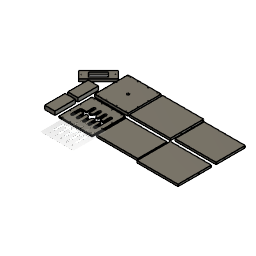
H shifeter (Autodesk Fusion 360 design; units mm, degrees)
part number: 2026-02-17-17-36-58-814
Autodesk Fusion 360 part; units mm, degrees
sketch "Sketch2" plane through (0, 0, 0) normal (0, 1, 0) x (1, 0, 0)
  line L0 (0, 65) -> (-65, 65)
  line L1 (-65, 65) -> (65, 65)
  line L2 (65, 65) -> (65, -65)
  line L3 (65, -65) -> (-65, -65)
  line L4 (-65, -65) -> (-65, 65)
  circle A0 centre (0, 0) radius 4.5
  circle A1 centre (-61, -63) radius 1
  circle A2 centre (-61, 61) radius 1
  circle A3 centre (-61, 17) radius 1
  circle A4 centre (-61, -23) radius 1
  line L5 (100, -65) -> (108, -65)
  line L6 (108, -65) -> (108, 65)
  line L7 (108, 65) -> (100, 65)
  line L8 (100, 65) -> (100, -65)
  line L9 (104, -64) -> (104, -63)
  line L10 (104, -63) -> (103, -63)
  circle A5 centre (104, -63) radius 1
  circle A6 centre (104, -23) radius 1
  circle A7 centre (104, 17) radius 1
  circle A8 centre (104, 61) radius 1
  line L11 (108, -65) -> (108, 65)
  line L12 (100, 65) -> (100, -65)
  line L13 (108, -65) -> (108, 65)
  line L14 (108, -65) -> (108, 65)
  circle A9 centre (104, -63) radius 1
  line L15 (104, -64) -> (104, -63)
  line L16 (100, -65) -> (108, -65)
  circle A10 centre (104, 61) radius 1
  line L17 (100, 65) -> (100, -65)
  circle A11 centre (104, -23) radius 1
  circle A12 centre (104, 17) radius 1
  line L18 (108, 65) -> (100, 65)
  line L19 (100, 65) -> (100, -65)
  line L20 (198, -57) -> (198, 57)
  line L21 (194, 52) -> (194, 54)
  line L22 (194, 52) -> (194, 54)
  line L23 (194, 52) -> (194, 53)
  line L24 (190, 57) -> (190, -57)
  line L25 (198, -57) -> (198, 57)
  line L26 (190, 57) -> (190, -57)
  line L27 (190, 57) -> (190, -57)
  circle A13 centre (61, -63) radius 1
  line L28 (65, -65) -> (65, 65)
  line L29 (65, -65) -> (65, 65)
  circle A14 centre (61, -63) radius 1
  line L30 (65, -65) -> (65, 65)
  line L31 (61, -65) -> (61, -63)
  circle A15 centre (61, -23) radius 1
  circle A16 centre (61, -23) radius 1
  line L32 (61, -63) -> (60, -63)
  line L33 (65, -65) -> (65, 65)
  line L34 (57, -65) -> (65, -65)
  circle A17 centre (61, 17) radius 1
  line L35 (61, -65) -> (61, -63)
  line L36 (61, -63) -> (60, -63)
  line L37 (57, -65) -> (65, -65)
  line L38 (65, 65) -> (57, 65)
  line L39 (65, 65) -> (57, 65)
  circle A18 centre (61, 61) radius 1
  circle A19 centre (61, 17) radius 1
  circle A20 centre (61, 61) radius 1
  line L40 (65, 57) -> (65, 65)
  circle A21 centre (17, 61) radius 1
  line L41 (-65, 65) -> (-65, 57)
  circle A22 centre (17, 61) radius 1
  circle A23 centre (61, 61) radius 1
  line L42 (65, 57) -> (65, 65)
  line L43 (-65, 65) -> (-65, 57)
  line L44 (65, 65) -> (-65, 65)
  line L45 (65, 65) -> (-65, 65)
  line L46 (65, 65) -> (-65, 65)
  line L47 (65, 65) -> (-65, 65)
  circle A24 centre (-23, 61) radius 1
  circle A25 centre (-23, 61) radius 1
  circle A26 centre (53, 61) radius 1
  line L48 (190, 57) -> (198, 57)
  line L49 (194, 54) -> (194, 53)
  circle A27 centre (194, 53) radius 1
  line L50 (190, -57) -> (198, -57)
  line L51 (190, 57) -> (190, -57)
  line L52 (194, -54) -> (194, -52)
  line L53 (194, -54) -> (194, -53)
  circle A28 centre (194, -53) radius 1
  circle A29 centre (-53, 61) radius 1
  circle A30 centre (194, -23) radius 1
  line L54 (194, -23) -> (194, -22)
  line L55 (194, 52) -> (194, 53)
  line L56 (194, 54) -> (194, 52)
  line L57 (194, -54) -> (194, -52)
  line L58 (194, -24) -> (194, -23)
  line L59 (194, -53) -> (194, -52)
  line L60 (194, -24) -> (194, -23)
  line L61 (194, -22) -> (194, -24)
  line L62 (194, -52) -> (194, -54)
  circle A31 centre (194, 17) radius 1
  line L63 (194, -23) -> (194, -22)
  line L64 (194, 16) -> (194, 17)
  circle A32 centre (234, 53) radius 1
  line L65 (238, -57) -> (238, 57)
  circle A33 centre (234, 17) radius 1
  line L66 (234, 52) -> (234, 53)
  line L67 (234, -54) -> (234, -52)
  circle A34 centre (234, -53) radius 1
  line L68 (234, -54) -> (234, -53)
  line L69 (234, -22) -> (234, -24)
  line L70 (234, -23) -> (234, -22)
  line L71 (234, -52) -> (234, -54)
  line L72 (234, 52) -> (234, 53)
  line L73 (234, 16) -> (234, 17)
  line L74 (234, -54) -> (234, -52)
  line L75 (234, -24) -> (234, -23)
  line L76 (234, -24) -> (234, -23)
  line L77 (230, 57) -> (230, -57)
  line L78 (230, -57) -> (238, -57)
  circle A35 centre (234, -23) radius 1
  line L79 (234, -23) -> (234, -22)
  line L80 (234, 54) -> (234, 53)
  line L81 (234, -53) -> (234, -52)
  line L82 (238, -57) -> (238, 57)
  line L83 (234, 52) -> (234, 54)
  line L84 (234, 54) -> (234, 52)
  line L85 (230, 57) -> (238, 57)
  line L86 (234, 52) -> (234, 54)
  line L87 (230, 57) -> (230, -57)
  line L88 (230, 57) -> (230, -57)
  line L89 (230, 57) -> (230, -57)
  line L90 (-24, -61) -> (-23, -61)
  line L91 (-24, -61) -> (-23, -61)
  line L92 (-52, -61) -> (-54, -61)
  line L93 (-22, -61) -> (-24, -61)
  line L94 (-23, -61) -> (-22, -61)
  circle A36 centre (-23, -61) radius 1
  line L95 (-23, -61) -> (-22, -61)
  line L96 (-54, -61) -> (-53, -61)
  circle A37 centre (17, -61) radius 1
  line L97 (52, -61) -> (53, -61)
  line L98 (52, -61) -> (54, -61)
  line L99 (-53, -61) -> (-52, -61)
  line L100 (52, -61) -> (53, -61)
  circle A38 centre (53, -61) radius 1
  line L101 (54, -61) -> (53, -61)
  line L102 (52, -61) -> (54, -61)
  line L103 (54, -61) -> (52, -61)
  line L104 (-54, -61) -> (-52, -61)
  line L105 (-54, -61) -> (-52, -61)
  circle A39 centre (-53, -61) radius 1
  line L106 (16, -61) -> (17, -61)
  line L107 (-61, -63) -> (-61, -62)
  line L108 (-61, -24) -> (-61, -23)
  line L109 (-61, -23) -> (-61, -22)
  line L110 (-61, 16) -> (-61, 17)
  line L111 (-61, 17) -> (-61, 18)
  line L112 (-61, 60) -> (-61, 61)
  line L113 (-24, 61) -> (-23, 61)
  line L114 (-24, 61) -> (-23, 61)
  line L115 (-62, 61) -> (-60, 61)
  line L116 (-57, 61) -> (-52, 61)
  line L117 (-62, 61) -> (-60, 61)
  line L118 (-54, 61) -> (-52, 61)
  line L119 (-23, 61) -> (-22, 61)
  line L120 (16, 61) -> (17, 61)
  line L121 (-23, 61) -> (-22, 61)
  line L122 (16, 61) -> (17, 61)
  line L123 (17, 61) -> (18, 61)
  line L124 (17, 61) -> (18, 61)
  line L125 (17, 61) -> (18, 61)
  line L126 (17, 61) -> (18, 61)
  line L127 (60, 61) -> (61, 61)
  line L128 (52, 61) -> (54, 61)
  line L129 (60, 61) -> (61, 61)
  line L130 (52, 61) -> (54, 61)
  line L131 (60, 61) -> (61, 61)
  line L132 (52, 61) -> (54, 61)
  line L133 (60, 61) -> (61, 61)
  line L134 (61, 17) -> (61, 18)
  line L135 (61, 60) -> (61, 61)
  line L136 (61, 17) -> (61, 18)
  line L137 (61, 60) -> (61, 61)
  line L138 (61, 17) -> (61, 18)
  line L139 (61, 60) -> (61, 61)
  line L140 (61, 17) -> (61, 18)
  line L141 (61, 60) -> (61, 61)
  line L142 (61, -23) -> (61, -22)
  line L143 (61, 16) -> (61, 17)
  line L144 (61, -23) -> (61, -22)
  line L145 (61, 16) -> (61, 17)
  line L146 (61, -63) -> (61, -62)
  line L147 (61, -24) -> (61, -23)
  line L148 (61, -63) -> (61, -62)
  line L149 (61, -24) -> (61, -23)
  line L150 (104, -23) -> (104, -22)
  line L151 (104, 16) -> (104, 17)
  line L152 (104, -63) -> (104, -62)
  line L153 (104, -24) -> (104, -23)
  line L154 (104, -23) -> (104, -22)
  line L155 (104, 16) -> (104, 17)
  line L156 (104, -63) -> (104, -62)
  line L157 (104, -24) -> (104, -23)
  line L158 (104, 17) -> (104, 18)
  line L159 (104, 60) -> (104, 61)
  line L160 (104, 17) -> (104, 18)
  line L161 (104, 60) -> (104, 61)
  line L162 (104, 17) -> (104, 18)
  line L163 (104, 60) -> (104, 61)
  line L164 (104, 17) -> (104, 18)
  line L165 (104, 60) -> (104, 61)
  circle A40 centre (134, -23) radius 1
  line L166 (138, -65) -> (138, 65)
  line L167 (138, -65) -> (138, 65)
  line L168 (138, -65) -> (138, 65)
  line L169 (134, -24) -> (134, -23)
  line L170 (134, -23) -> (134, -22)
  line L171 (130, 65) -> (130, -65)
  line L172 (138, -65) -> (138, 65)
  line L173 (130, 65) -> (130, -65)
  circle A41 centre (134, 61) radius 1
  line L174 (134, 17) -> (134, 18)
  line L175 (138, 65) -> (130, 65)
  line L176 (134, 60) -> (134, 61)
  line L177 (134, 17) -> (134, 18)
  circle A42 centre (134, 17) radius 1
  line L178 (134, 17) -> (134, 18)
  circle A43 centre (134, 61) radius 1
  line L179 (134, 60) -> (134, 61)
  circle A44 centre (134, 17) radius 1
  line L180 (134, 60) -> (134, 61)
  line L181 (134, 60) -> (134, 61)
  line L182 (134, 16) -> (134, 17)
  line L183 (138, 65) -> (130, 65)
  circle A45 centre (134, -63) radius 1
  line L184 (130, 65) -> (130, -65)
  line L185 (130, 65) -> (130, -65)
  line L186 (134, -63) -> (133, -63)
  line L187 (134, 17) -> (134, 18)
  line L188 (134, -64) -> (134, -63)
  line L189 (134, -63) -> (134, -62)
  circle A46 centre (134, -63) radius 1
  line L190 (130, -65) -> (138, -65)
  line L191 (134, -64) -> (134, -63)
  line L192 (134, -63) -> (134, -62)
  line L193 (134, -63) -> (133, -63)
  line L194 (134, 16) -> (134, 17)
  line L195 (130, -65) -> (138, -65)
  circle A47 centre (134, -23) radius 1
  line L196 (134, -24) -> (134, -23)
  line L197 (134, -23) -> (134, -22)
  line L198 (-57, -189) -> (-52, -189)
  line L199 (16, -189) -> (17, -189)
  line L200 (-61, -234) -> (-61, -233)
  line L201 (-24, -189) -> (-23, -189)
  line L202 (-61, -233) -> (-61, -232)
  line L203 (-65, -185) -> (-65, -193)
  line L204 (-65, -185) -> (-65, -193)
  line L205 (-62, -189) -> (-60, -189)
  line L206 (-61, -190) -> (-61, -189)
  line L207 (-23, -189) -> (-22, -189)
  circle A48 centre (17, -189) radius 1
  line L208 (-62, -189) -> (-60, -189)
  circle A49 centre (-23, -189) radius 1
  line L209 (17, -189) -> (18, -189)
  line L210 (17, -189) -> (18, -189)
  line L211 (0, -185) -> (-65, -185)
  line L212 (-23, -189) -> (-22, -189)
  line L213 (17, -189) -> (18, -189)
  circle A50 centre (17, -189) radius 1
  line L214 (-54, -189) -> (-52, -189)
  line L215 (-24, -189) -> (-23, -189)
  line L216 (17, -189) -> (18, -189)
  line L217 (65, -185) -> (-65, -185)
  line L218 (-65, -185) -> (65, -185)
  line L219 (65, -185) -> (-65, -185)
  line L220 (65, -315) -> (-65, -315)
  line L221 (65, -185) -> (-65, -185)
  line L222 (65, -185) -> (-65, -185)
  line L223 (-65, -315) -> (-65, -185)
  circle A51 centre (-23, -311) radius 1
  line L224 (65, -315) -> (65, -185)
  line L225 (16, -311) -> (17, -311)
  line L226 (-53, -311) -> (-52, -311)
  line L227 (-52, -311) -> (-54, -311)
  line L228 (-23, -311) -> (-22, -311)
  line L229 (-24, -311) -> (-23, -311)
  line L230 (65, -185) -> (65, -315)
  line L231 (-22, -311) -> (-24, -311)
  circle A52 centre (-53, -311) radius 1
  line L232 (-61, -274) -> (-61, -273)
  circle A53 centre (-61, -233) radius 1
  line L233 (-54, -311) -> (-53, -311)
  circle A54 centre (-53, -189) radius 1
  circle A55 centre (-61, -273) radius 1
  line L234 (16, -189) -> (17, -189)
  circle A56 centre (-61, -313) radius 1
  line L235 (-23, -311) -> (-22, -311)
  line L236 (-61, -273) -> (-61, -272)
  line L237 (-61, -313) -> (-61, -312)
  line L238 (-54, -311) -> (-52, -311)
  circle A57 centre (17, -311) radius 1
  line L239 (-54, -311) -> (-52, -311)
  line L240 (-24, -311) -> (-23, -311)
  circle A58 centre (-23, -189) radius 1
  circle A59 centre (-61, -189) radius 1
  line L241 (65, -315) -> (65, -185)
  circle A60 centre (61, -313) radius 1
  line L242 (57, -315) -> (65, -315)
  line L243 (52, -311) -> (54, -311)
  line L244 (61, -313) -> (60, -313)
  line L245 (52, -311) -> (54, -311)
  line L246 (61, -313) -> (60, -313)
  line L247 (54, -311) -> (52, -311)
  line L248 (65, -315) -> (65, -185)
  circle A61 centre (53, -311) radius 1
  line L249 (65, -315) -> (65, -185)
  line L250 (65, -193) -> (65, -185)
  line L251 (61, -274) -> (61, -273)
  line L252 (61, -233) -> (61, -232)
  circle A62 centre (61, -273) radius 1
  circle A63 centre (61, -313) radius 1
  circle A64 centre (61, -273) radius 1
  circle A65 centre (61, -189) radius 1
  circle A66 centre (61, -233) radius 1
  line L253 (52, -189) -> (54, -189)
  line L254 (61, -234) -> (61, -233)
  line L255 (61, -190) -> (61, -189)
  line L256 (52, -189) -> (54, -189)
  line L257 (65, -193) -> (65, -185)
  line L258 (61, -274) -> (61, -273)
  line L259 (61, -313) -> (61, -312)
  line L260 (57, -315) -> (65, -315)
  line L261 (61, -233) -> (61, -232)
  line L262 (54, -311) -> (53, -311)
  line L263 (61, -233) -> (61, -232)
  line L264 (61, -273) -> (61, -272)
  line L265 (52, -189) -> (54, -189)
  circle A67 centre (61, -233) radius 1
  line L266 (65, -185) -> (57, -185)
  line L267 (52, -311) -> (53, -311)
  line L268 (61, -315) -> (61, -313)
  line L269 (61, -315) -> (61, -313)
  line L270 (65, -185) -> (57, -185)
  line L271 (52, -311) -> (53, -311)
  line L272 (61, -313) -> (61, -312)
  line L273 (60, -189) -> (61, -189)
  line L274 (60, -189) -> (61, -189)
  circle A68 centre (53, -189) radius 1
  circle A69 centre (61, -189) radius 1
  line L275 (61, -273) -> (61, -272)
  line L276 (60, -189) -> (61, -189)
  circle A70 centre (61, -189) radius 1
  line L277 (61, -233) -> (61, -232)
  line L278 (61, -190) -> (61, -189)
  line L279 (61, -190) -> (61, -189)
  line L280 (60, -189) -> (61, -189)
  line L281 (61, -190) -> (61, -189)
  line L282 (61, -234) -> (61, -233)
  arc A71 (17.3155, -282.4056) -> (26.3155, -282.4056) centre (21.8155, -282.4056) ccw
  line L283 (39, -245.5) -> (26.3155, -245.5)
  line L284 (26.3155, -254.5058) -> (39, -254.5058)
  arc A72 (48, -220) -> (39, -220) centre (43.5, -220) ccw
  arc A73 (26.3155, -220) -> (17.3155, -220) centre (21.8155, -220) ccw
  arc A74 (39, -282.4056) -> (48, -282.4056) centre (43.5, -282.4056) ccw
  line L285 (5.3081, -282.4056) -> (5.3081, -259.4163)
  arc A75 (-16.9818, -220) -> (-25.9818, -220) centre (-21.4818, -220) ccw
  line L286 (-4.241, -240.0573) -> (-4.241, -220)
  line L287 (39, -254.5058) -> (39, -282.4056)
  arc A76 (4.759, -220) -> (-4.241, -220) centre (0.259, -220) ccw
  line L288 (-18, -282.6168) -> (-18, -254.8691)
  line L289 (17.3155, -254.5058) -> (17.3155, -282.4056)
  line L290 (-27, -255) -> (-27, -282.6168)
  arc A77 (-41.9906, -245.6112) -> (-49, -251.5257) centre (-43, -251.5257) ccw
  line L291 (48, -254.5058) -> (48, -220)
  line L292 (39, -220) -> (39, -245.5)
  arc A78 (-49, -282.6168) -> (-40, -282.6168) centre (-44.5, -282.6168) ccw
  line L293 (-16.9818, -220) -> (-16.9818, -245.8691)
  arc A79 (5.3081, -259.4163) -> (9.8255, -254.5058) centre (0, -250) ccw
  line L294 (26.3155, -282.4056) -> (26.3155, -254.5058)
  line L295 (9.8255, -254.5058) -> (17.3155, -254.5058)
  arc A80 (-4.241, -240.0573) -> (-9.9889, -245.8691) centre (0, -250) ccw
  line L296 (-3.6919, -260.1594) -> (-3.6919, -282.4056)
  line L297 (-49, -282.6168) -> (-49, -251.5257)
  line L298 (17.3155, -220) -> (17.3155, -245.4147)
  line L299 (-16.9818, -245.8691) -> (-9.9889, -245.8691)
  line L300 (-8.9707, -254.8691) -> (-18, -254.8691)
  arc A81 (-27, -282.6168) -> (-18, -282.6168) centre (-22.5, -282.6168) ccw
  line L301 (-40, -255) -> (-40, -282.6168)
  line L302 (17.3155, -245.4147) -> (9.7887, -245.4147)
  line L303 (48, -282.4056) -> (48, -254.5058)
  line L304 (26.3155, -245.5) -> (26.3155, -220)
  line L305 (-27, -255) -> (-40, -255)
  arc A82 (-9.6507, -254.8691) -> (-3.6919, -260.1594) centre (0, -250) ccw
  line L306 (-25.9818, -245.6112) -> (-25.9818, -220)
  arc A83 (-3.6919, -282.4056) -> (5.3081, -282.4056) centre (0.8081, -282.4056) ccw
  arc A84 (9.7887, -245.4147) -> (4.759, -240.2946) centre (0, -250) ccw
  line L307 (4.759, -220) -> (4.759, -241)
  line L308 (-41.9906, -245.6112) -> (-25.9818, -245.6112)
  dimension "d5" = 130
  dimension "d6" = 130
  dimension "d11" = 9
  dimension "d17" = 40
  dimension "d18" = 40
  dimension "d19" = 44
  dimension "d20" = 2
  dimension "d21" = 2
  dimension "d22" = 2
  dimension "d23" = 8
  dimension "d24" = 130
  dimension "d25" = 40
  dimension "d26" = 40
  dimension "d27" = 44
  dimension "d28" = 2
  dimension "d29" = 2
  dimension "d30" = 2
  dimension "d31" = 2
  dimension "d32" = 8
  dimension "d33" = 130
  dimension "d34" = 44
  dimension "d45" = 8
  dimension "d46" = 130
  dimension "d47" = 40
  dimension "d48" = 40
  dimension "d49" = 44
  dimension "d50" = 2
  dimension "d51" = 2
  dimension "d52" = 2
  dimension "d53" = 2
  dimension "d54" = 8
  dimension "d55" = 130
  dimension "d56" = 44
  dimension "d111" = 8
  dimension "d112" = 130
  dimension "d113" = 40
  dimension "d114" = 40
  dimension "d115" = 44
  dimension "d116" = 2
  dimension "d117" = 2
  dimension "d118" = 2
  dimension "d119" = 2
  dimension "d122" = 44
  dimension "d123" = 8
  dimension "d124" = 130
  dimension "d125" = 40
  dimension "d126" = 40
  dimension "d127" = 44
  dimension "d128" = 2
  dimension "d129" = 2
  dimension "d130" = 2
  dimension "d131" = 2
  dimension "d134" = 44
  dimension "d135" = 8
  dimension "d136" = 130
  dimension "d138" = 40
  dimension "d139" = 44
  dimension "d141" = 2
  dimension "d142" = 2
  dimension "d143" = 2
  dimension "d145" = 130
  dimension "d146" = 44
  dimension "d147" = 8
  dimension "d148" = 130
  dimension "d150" = 40
  dimension "d151" = 44
  dimension "d153" = 2
  dimension "d154" = 2
  dimension "d157" = 130
  dimension "d158" = 44
  dimension "d159" = 2
  dimension "d162" = 2
  dimension "d164" = 2
  dimension "d166" = 2
  dimension "d167" = 30
  dimension "d168" = 2
  dimension "d171" = 40
  dimension "d172" = 2
  dimension "d173" = 2
  dimension "d174" = 2
  dimension "d175" = 30
  dimension "d176" = 2
  dimension "d177" = 40
  dimension "d178" = 2
  dimension "d179" = 2
  dimension "d180" = 2
  dimension "d181" = 30
  dimension "d182" = 2
  dimension "d183" = 40
  dimension "d184" = 2
  dimension "d185" = 8
  dimension "d186" = 130
  dimension "d187" = 40
  dimension "d188" = 40
  dimension "d189" = 44
  dimension "d190" = 2
  dimension "d191" = 2
  dimension "d192" = 2
  dimension "d193" = 2
  dimension "d194" = 8
  dimension "d195" = 130
  dimension "d196" = 44
  dimension "d197" = 8
  dimension "d198" = 130
  dimension "d199" = 40
  dimension "d200" = 40
  dimension "d201" = 44
  dimension "d202" = 2
  dimension "d203" = 2
  dimension "d204" = 2
  dimension "d205" = 2
  dimension "d206" = 8
  dimension "d207" = 130
  dimension "d208" = 44
  dimension "d209" = 130
  dimension "d210" = 130
  dimension "d212" = 40
  dimension "d213" = 40
  dimension "d214" = 44
  dimension "d215" = 2
  dimension "d216" = 2
  dimension "d217" = 2
  dimension "d218" = 8
  dimension "d219" = 130
  dimension "d220" = 40
  dimension "d221" = 40
  dimension "d222" = 44
  dimension "d223" = 2
  dimension "d224" = 2
  dimension "d225" = 2
  dimension "d226" = 2
  dimension "d227" = 44
  dimension "d228" = 8
  dimension "d229" = 130
  dimension "d230" = 40
  dimension "d231" = 40
  dimension "d232" = 44
  dimension "d233" = 2
  dimension "d234" = 2
  dimension "d235" = 2
  dimension "d236" = 2
  dimension "d237" = 44
  dimension "d238" = 8
  dimension "d239" = 130
  dimension "d240" = 40
  dimension "d241" = 44
  dimension "d242" = 2
  dimension "d243" = 2
  dimension "d244" = 2
  dimension "d245" = 130
  dimension "d246" = 44
  dimension "d247" = 8
  dimension "d248" = 130
  dimension "d249" = 40
  dimension "d250" = 44
  dimension "d251" = 2
  dimension "d252" = 2
  dimension "d253" = 130
  dimension "d254" = 44
  dimension "d255" = 2
  dimension "d256" = 2
  dimension "d257" = 2
  dimension "d258" = 2
  dimension "d259" = 30
  dimension "d260" = 2
  dimension "d261" = 40
  dimension "d262" = 2
  dimension "d274" = 9
  dimension "d275" = 9
  dimension "d276" = 9
  dimension "d277" = 9
  dimension "d278" = 9
  dimension "d279" = 9
  dimension "d280" = 25.5
  dimension "d281" = 9
  dimension "d282" = 9
  dimension "d283" = 9
  constraint horizontal L1
  constraint vertical L2
  constraint horizontal L3
  constraint vertical L4
  constraint coincident A0.centre origin
  constraint coincident A1.centre L107.start
  constraint parallel L4 L107
  constraint parallel L108 L109
  constraint parallel L110 L111
  constraint coincident A2.centre L112.end
  constraint coincident A3.centre L110.end
  constraint coincident A4.centre L108.end
  constraint horizontal L5
  constraint vertical L6
  constraint horizontal L7
  constraint vertical L8
  constraint perpendicular L5 L9
  constraint perpendicular L8 L10
  constraint perpendicular L10 L156
  constraint perpendicular L10 L150
  constraint perpendicular L10 L162
  constraint coincident L9.end L10.start
  constraint coincident A6.centre A11.centre
  constraint coincident A7.centre A12.centre
  constraint coincident A8.centre A10.centre
  constraint vertical L11
  constraint vertical L12
  constraint horizontal L16
  constraint vertical L13
  constraint horizontal L18
  constraint vertical L19
  constraint perpendicular L15 L16
  constraint vertical L14
  constraint vertical L17
  constraint vertical L25
  constraint vertical L51
  constraint vertical L24
  constraint vertical L27
  constraint vertical L20
  constraint vertical L26
  constraint horizontal L37
  constraint vertical L33
  constraint horizontal L39
  constraint midpoint L31.start L37
  constraint perpendicular L31 L37
  constraint perpendicular L36 L148
  constraint perpendicular L36 L142
  constraint perpendicular L36 L140
  constraint coincident A13.centre A14.centre
  constraint coincident A15.centre A16.centre
  constraint coincident A17.centre A19.centre
  constraint coincident A18.centre A20.centre
  constraint vertical L30
  constraint horizontal L34
  constraint vertical L29
  constraint horizontal L38
  constraint midpoint L31.start L34
  constraint perpendicular L34 L35
  constraint perpendicular L32 L146
  constraint perpendicular L32 L144
  constraint perpendicular L32 L134
  constraint vertical L28
  constraint coincident A24.centre A25.centre
  constraint coincident A21.centre A22.centre
  constraint coincident A26.centre L127
  constraint perpendicular L20 L48
  constraint parallel L22 L49
  constraint coincident L23.end L49.end
  constraint parallel L23 L49
  constraint coincident A27 L21.start
  constraint perpendicular L25 L50
  constraint coincident L53.end L62
  constraint coincident L53.end A28.centre
  constraint coincident A29.centre L118
  constraint coincident A30.centre L54.start
  constraint parallel L54 L61
  constraint parallel L55 L56
  constraint coincident A30 L54.end
  constraint collinear L56 L61
  constraint coincident A27 L21.end
  constraint coincident A28 L52.end
  constraint coincident A30 L58.start
  constraint collinear L57 L58
  constraint collinear L59 L60
  constraint collinear L61 L62
  constraint coincident A28 L52.start
  constraint coincident A31.centre L64.end
  constraint coincident A31 L64.start
  constraint collinear L63 L64
  constraint vertical L82
  constraint vertical L89
  constraint vertical L87
  constraint vertical L77
  constraint vertical L65
  constraint vertical L88
  constraint perpendicular L65 L85
  constraint parallel L80 L86
  constraint coincident A32.centre L66.end
  constraint parallel L72 L80
  constraint coincident L66.start A32
  constraint perpendicular L78 L82
  constraint coincident A34.centre L71
  constraint coincident A34.centre L68.end
  constraint coincident L70.start L75.end
  constraint parallel L69 L70
  constraint parallel L66 L84
  constraint coincident L69.start A35
  constraint collinear L69 L84
  constraint coincident L80.start A32
  constraint coincident L67.end A34
  constraint coincident L69.end A35
  constraint collinear L74 L76
  constraint collinear L75 L81
  constraint collinear L69 L71
  constraint coincident L67.start A34
  constraint coincident A33.centre L73.end
  constraint coincident L73.start A33
  constraint collinear L73 L79
  constraint parallel L98 L101
  constraint coincident L97.end L100.end
  constraint parallel L100 L101
  constraint coincident L97.start A38
  constraint coincident L96.end L92
  constraint coincident L96.end L99.start
  constraint coincident L90.end L91.end
  constraint parallel L93 L95
  constraint parallel L97 L103
  constraint coincident L93.start A36
  constraint collinear L93 L103
  constraint coincident L98.end A38
  constraint coincident L92.start A39
  constraint coincident L90.start A36
  constraint collinear L91 L105
  constraint collinear L90 L99
  constraint collinear L92 L93
  constraint coincident L92.end A39
  constraint coincident A37.centre L106.end
  constraint coincident L106.start A37
  constraint collinear L94 L106
  constraint coincident A1 L107.end
  constraint coincident A4 L108.start
  constraint collinear L107 L108
  constraint coincident A4 L109.end
  constraint coincident A3 L110.start
  constraint collinear L109 L110
  constraint coincident A3 L111.end
  constraint collinear L111 L112
  constraint coincident A29 L116.end
  constraint coincident A24 L113.start
  constraint collinear L113 L116
  constraint collinear L114 L118
  constraint coincident A2 L115.end
  constraint collinear L115 L116
  constraint collinear L117 L118
  constraint coincident A29 L118.start
  constraint coincident A2 L112.start
  constraint coincident A2 L115.start
  constraint coincident A24 L119.end
  constraint collinear L119 L120
  constraint coincident A21 L120.start
  constraint collinear L121 L122
  constraint coincident A21 L123.end
  constraint coincident A26 L128.start
  constraint collinear L123 L132
  constraint collinear L124 L128
  constraint collinear L125 L130
  constraint collinear L126 L127
  constraint coincident A26 L128.end
  constraint collinear L128 L129
  constraint coincident A18 L127.start
  constraint collinear L130 L131
  constraint collinear L132 L133
  constraint coincident A17 L134.end
  constraint collinear L134 L135
  constraint coincident A18 L135.start
  constraint collinear L136 L137
  constraint collinear L138 L139
  constraint collinear L140 L141
  constraint coincident A15 L142.end
  constraint coincident A17 L143.start
  constraint collinear L142 L143
  constraint collinear L144 L145
  constraint coincident A13 L146.end
  constraint coincident A15 L147.start
  constraint collinear L146 L147
  constraint collinear L148 L149
  constraint coincident A13 L32.end
  constraint coincident A6 L150.end
  constraint coincident A7 L151.start
  constraint collinear L150 L151
  constraint coincident A5 L152.end
  constraint coincident A6 L153.start
  constraint collinear L152 L153
  constraint collinear L154 L155
  constraint collinear L156 L157
  constraint coincident A7 L158.end
  constraint coincident A8 L159.start
  constraint collinear L158 L159
  constraint collinear L160 L161
  constraint collinear L162 L163
  constraint collinear L164 L165
  constraint horizontal L190
  constraint vertical L168
  constraint horizontal L183
  constraint vertical L185
  constraint perpendicular L190 L191
  constraint perpendicular L185 L193
  constraint perpendicular L189 L193
  constraint perpendicular L170 L193
  constraint perpendicular L177 L193
  constraint coincident A45.centre L186.start
  constraint coincident A40.centre L169.end
  constraint coincident L174.start L177.start
  constraint coincident A41.centre L176.end
  constraint vertical L167
  constraint vertical L173
  constraint horizontal L195
  constraint vertical L166
  constraint horizontal L175
  constraint vertical L184
  constraint perpendicular L188 L195
  constraint perpendicular L184 L186
  constraint perpendicular L186 L192
  constraint perpendicular L186 L197
  constraint perpendicular L174 L186
  constraint vertical L172
  constraint vertical L171
  constraint coincident L170.end A47
  constraint coincident L182.start A44
  constraint collinear L170 L182
  constraint coincident L189.end A45
  constraint coincident L169.start A47
  constraint collinear L169 L192
  constraint collinear L194 L197
  constraint collinear L189 L196
  constraint coincident L174.end A44
  constraint coincident L176.start A41
  constraint collinear L181 L187
  constraint collinear L174 L179
  constraint collinear L177 L180
  constraint collinear L176 L178
  constraint horizontal L218
  constraint vertical L230
  constraint horizontal L220
  constraint vertical L223
  constraint coincident A56.centre L237.start
  constraint parallel L223 L237
  constraint parallel L232 L236
  constraint parallel L200 L202
  constraint coincident L206.end A59.centre
  constraint coincident L200.end L202.start
  constraint coincident L232.end A55.centre
  constraint horizontal L242
  constraint vertical L249
  constraint horizontal L266
  constraint midpoint L268.start L242
  constraint perpendicular L242 L268
  constraint perpendicular L244 L272
  constraint perpendicular L244 L264
  constraint perpendicular L244 L277
  constraint coincident A60.centre L244.start
  constraint coincident L251.end A62.centre
  constraint coincident L252.start A66.centre
  constraint coincident A65.centre L255.end
  constraint vertical L241
  constraint horizontal L260
  constraint vertical L224
  constraint horizontal L270
  constraint midpoint L268.start L260
  constraint perpendicular L260 L269
  constraint perpendicular L246 L259
  constraint perpendicular L246 L275
  constraint perpendicular L246 L252
  constraint vertical L248
  constraint coincident L201.end L207.start
  constraint coincident L199.end A48.centre
  constraint coincident A68.centre L273
  constraint coincident A54.centre L214
  constraint parallel L245 L262
  constraint coincident A61.centre L262.end
  constraint parallel L262 L271
  constraint coincident L243.start A61
  constraint coincident L226.start L227
  constraint coincident L226.start A52.centre
  constraint coincident A51.centre L228.start
  constraint parallel L228 L231
  constraint parallel L247 L267
  constraint coincident L228.end A51
  constraint collinear L231 L247
  constraint coincident L243.end A61
  constraint coincident L226.end A52
  constraint coincident L229.start A51
  constraint collinear L229 L239
  constraint collinear L226 L240
  constraint collinear L227 L231
  constraint coincident L227.end A52
  constraint coincident L225.end A57.centre
  constraint coincident L225.start A57
  constraint collinear L225 L235
  constraint coincident L237.end A56
  constraint coincident L232.start A55
  constraint collinear L232 L237
  constraint coincident L236.end A55
  constraint coincident L200.start A53
  constraint collinear L200 L236
  constraint coincident L202.end A53
  constraint collinear L202 L206
  constraint coincident L198.end A54
  constraint coincident L201.start A49
  constraint collinear L198 L215
  constraint collinear L201 L214
  constraint coincident L205.end A59
  constraint collinear L198 L205
  constraint collinear L208 L214
  constraint coincident L214.start A54
  constraint coincident L206.start A59
  constraint coincident L205.start A59
  constraint coincident L207.end A49
  constraint collinear L207 L234
  constraint coincident L199.start A50
  constraint collinear L199 L212
  constraint coincident L209.end A50
  constraint coincident L253.start A68
  constraint collinear L213 L265
  constraint collinear L210 L253
  constraint collinear L209 L256
  constraint collinear L216 L273
  constraint coincident L253.end A68
  constraint collinear L253 L274
  constraint coincident L273.start A69
  constraint collinear L256 L280
  constraint collinear L265 L276
  constraint coincident L252.end A66
  constraint collinear L252 L279
  constraint coincident L255.start A69
  constraint collinear L263 L278
  constraint collinear L255 L261
  constraint collinear L277 L281
  constraint coincident L264.end A64
  constraint coincident L254.start A66
  constraint collinear L264 L282
  constraint collinear L254 L275
  constraint coincident L259.end A63
  constraint coincident L251.start A64
  constraint collinear L258 L259
  constraint collinear L251 L272
  constraint coincident L244.end A63
  constraint horizontal L300
  constraint perpendicular L288 L300
  constraint perpendicular L290 L305
  constraint perpendicular L301 L305
  constraint perpendicular L297 L308
  constraint perpendicular L306 L308
  constraint perpendicular L293 L299
  constraint tangent A77 L297
  constraint vertical L296
  constraint perpendicular L285 L295
  constraint perpendicular L289 L295
  constraint perpendicular L294 L295
  constraint perpendicular L284 L289
  constraint perpendicular L284 L287
  constraint perpendicular L284 L292
  constraint perpendicular L283 L292
  constraint perpendicular L292 L302
  constraint coincident A82.start L300
  constraint concentric A80 A82
  constraint concentric A79 A82
  constraint coincident A84.end L307
  constraint concentric A80 A84
  constraint tangent L288 A81
  constraint coincident A5 L10.end
  constraint coincident A5 L9.start
  constraint coincident A45 L186.end
  constraint coincident A45 L188.start
  measures "d5" distance of L0.end L1.end
  measures "d6" distance of L0.end L3.end
  measures "d11" diameter of A0
  measures "d17" distance of A1.centre A4.centre
  measures "d18" distance of A4.centre A3.centre
  measures "d19" distance of A3.centre A2.centre
  measures "d20" diameter of A2
  measures "d21" diameter of A3
  measures "d22" diameter of A4
  measures "d23" distance of L5.start L5.end
  measures "d24" distance of L5.start L7.end
  measures "d25" distance of L9.end A6.centre
  measures "d26" distance of A6.centre A7.centre
  measures "d27" distance of A7.centre A8.centre
  measures "d28" diameter of A5
  measures "d29" diameter of A6
  measures "d30" diameter of A7
  measures "d31" diameter of A8
  measures "d32" distance of L5.end L5.start
  measures "d33" distance of L7.end L5.start
  measures "d34" distance of A7.centre A8.centre
  measures "d45" distance of L5.end L5.start
  measures "d46" distance of L7.end L5.start
  measures "d47" distance of L9.end A6.centre
  measures "d48" distance of A7.centre A6.centre
  measures "d49" distance of A7.centre A8.centre
  measures "d50" diameter of A9
  measures "d51" diameter of A11
  measures "d52" diameter of A12
  measures "d53" diameter of A10
  measures "d54" distance of L5.end L5.start
  measures "d55" distance of L5.start L7.end
  measures "d56" distance of A8.centre A7.centre
  measures "d111" distance of L2.end L34.start
  measures "d112" distance of L38.end L34.start
  measures "d113" distance of A13.centre A15.centre
  measures "d114" distance of A17.centre A15.centre
  measures "d115" distance of A17.centre A18.centre
  measures "d116" diameter of A14
  measures "d117" diameter of A15
  measures "d118" diameter of A17
  measures "d119" diameter of A20
  measures "d122" distance of A18.centre A17.centre
  measures "d123" distance of L2.end L34.start
  measures "d124" distance of L38.end L34.start
  measures "d125" distance of A13.centre A15.centre
  measures "d126" distance of A17.centre A15.centre
  measures "d127" distance of A17.centre A18.centre
  measures "d128" diameter of A13
  measures "d129" diameter of A16
  measures "d130" diameter of A19
  measures "d131" diameter of A18
  measures "d134" distance of A18.centre A17.centre
  measures "d135" distance of L41.end L0.end
  measures "d136" distance of L1.end L0.end
  measures "d138" distance of A21.centre A24.centre
  measures "d139" distance of A21.centre A18.centre
  measures "d141" diameter of A25
  measures "d142" diameter of A22
  measures "d143" diameter of A23
  measures "d145" distance of L0.end L1.end
  measures "d146" distance of A18.centre A21.centre
  measures "d147" distance of L41.end L0.end
  measures "d148" distance of L1.end L0.end
  measures "d150" distance of A21.centre A24.centre
  measures "d151" distance of A21.centre A18.centre
  measures "d153" diameter of A24
  measures "d154" diameter of A21
  measures "d157" distance of L0.end L1.end
  measures "d158" distance of A18.centre A21.centre
  measures "d159" diameter of A26
  measures "d162" diameter of A27
  measures "d164" diameter of A28
  measures "d166" diameter of A29
  measures "d167" distance of A30.centre L53.end
  measures "d168" diameter of A30
  measures "d171" distance of A30.centre A31.centre
  measures "d172" diameter of A31
  measures "d173" diameter of A32
  measures "d174" diameter of A34
  measures "d175" distance of L70.start A34.centre
  measures "d176" diameter of A35
  measures "d177" distance of L70.start A33.centre
  measures "d178" diameter of A33
  measures "d179" diameter of A38
  measures "d180" diameter of A39
  measures "d181" distance of L90.end L96.end
  measures "d182" diameter of A36
  measures "d183" distance of L90.end A37.centre
  measures "d184" diameter of A37
  measures "d185" distance of L166.start L171.end
  measures "d186" distance of L171.start L171.end
  measures "d187" distance of A45.centre A40.centre
  measures "d188" distance of L174.start A40.centre
  measures "d189" distance of L174.start A41.centre
  measures "d190" diameter of A45
  measures "d191" diameter of A47
  measures "d192" diameter of A44
  measures "d193" diameter of A41
  measures "d194" distance of L166.start L171.end
  measures "d195" distance of L171.end L171.start
  measures "d196" distance of A41.centre L174.start
  measures "d197" distance of L166.start L171.end
  measures "d198" distance of L171.start L171.end
  measures "d199" distance of A45.centre A40.centre
  measures "d200" distance of L174.start A40.centre
  measures "d201" distance of L174.start A41.centre
  measures "d202" diameter of A46
  measures "d203" diameter of A40
  measures "d204" diameter of A42
  measures "d205" diameter of A43
  measures "d206" distance of L166.start L171.end
  measures "d207" distance of L171.end L171.start
  measures "d208" distance of A41.centre L174.start
  measures "d209" distance of L203.start L217.start
  measures "d210" distance of L220.end L203.start
  measures "d212" distance of A56.centre L232.end
  measures "d213" distance of L200.end L232.end
  measures "d214" distance of L206.end L200.end
  measures "d215" diameter of A59
  measures "d216" diameter of A53
  measures "d217" diameter of A55
  measures "d218" distance of L242.start L220.start
  measures "d219" distance of L242.start L266.end
  measures "d220" distance of L251.end A60.centre
  measures "d221" distance of L251.end L252.start
  measures "d222" distance of L252.start A65.centre
  measures "d223" diameter of A60
  measures "d224" diameter of A64
  measures "d225" diameter of A66
  measures "d226" diameter of A70
  measures "d227" distance of A65.centre L252.start
  measures "d228" distance of L242.start L220.start
  measures "d229" distance of L266.end L242.start
  measures "d230" distance of A60.centre L251.end
  measures "d231" distance of L252.start L251.end
  measures "d232" distance of A65.centre L252.start
  measures "d233" diameter of A63
  measures "d234" diameter of A62
  measures "d235" diameter of A67
  measures "d236" diameter of A69
  measures "d237" distance of A65.centre L252.start
  measures "d238" distance of L203.end L203.start
  measures "d239" distance of L217.start L203.start
  measures "d240" distance of L199.end L201.end
  measures "d241" distance of A65.centre L199.end
  measures "d242" diameter of A58
  measures "d243" diameter of A48
  measures "d244" diameter of A65
  measures "d245" distance of L203.start L217.start
  measures "d246" distance of A65.centre L199.end
  measures "d247" distance of L203.end L203.start
  measures "d248" distance of L217.start L203.start
  measures "d249" distance of L201.end L199.end
  measures "d250" distance of L199.end A65.centre
  measures "d251" diameter of A49
  measures "d252" diameter of A50
  measures "d253" distance of L217.start L203.start
  measures "d254" distance of L199.end A65.centre
  measures "d255" diameter of A68
  measures "d256" diameter of A54
  measures "d257" diameter of A61
  measures "d258" diameter of A52
  measures "d259" distance of A51.centre L226.start
  measures "d260" diameter of A51
  measures "d261" distance of L225.end A51.centre
  measures "d262" diameter of A57
  measures "d274" distance of A78.end A78.start
  measures "d275" distance of A75.start A75.end
  measures "d276" distance of L285.start L296.end
  measures "d277" distance of A71.end A71.start
  measures "d278" distance of A74.end A74.start
  measures "d279" distance of A72.end A72.start
  measures "d280" distance of A72.end L283.start
  measures "d281" distance of A73.end A73.start
  measures "d282" distance of L286.end A76.start
  measures "d283" diameter of A83
sketch "Sketch6" plane through (0, 0, 0) normal (0, 1, 0) x (1, 0, 0)
  line L0 (-145.6153, -170.4461) -> (-145.6153, -60.4461)
  line L1 (-145.6153, -60.4461) -> (-105.6153, -60.4461)
  line L2 (-105.6153, -60.4461) -> (-105.6153, -170.4461)
  line L3 (-170, -160) -> (-210, -160)
  line L4 (-210, -160) -> (-210, -145)
  line L5 (-210, -145) -> (-170, -145)
  line L6 (-170, -145) -> (-170, -160)
  line L7 (-170, -135) -> (-210, -135)
  line L8 (-210, -120) -> (-170, -120)
  line L9 (-170, -120) -> (-170, -135)
  line L10 (-210, -135) -> (-210, -120)
  line L11 (-105.6153, -155) -> (-105, -155)
  circle A0 centre (-125, -162.5) radius 1
  circle A1 centre (-125.6153, -67.9461) radius 1
  line L12 (-105.6153, -170.4461) -> (-145.6153, -170.4461)
  line L13 (-136.0595, -142.9461) -> (-113.3301, -142.9461)
  line L14 (-113.3301, -142.9461) -> (-113.3301, -87.9461)
  line L15 (-113.3301, -87.9461) -> (-136.0595, -87.9461)
  line L16 (-136.0595, -87.9461) -> (-136.0595, -142.9461)
  dimension "d284" = 40
  dimension "d285" = 110
  dimension "d286" = 40
  dimension "d287" = 15
  dimension "d289" = 40
  dimension "d290" = 15
  dimension "d294" = 2
  dimension "d296" = 2
  dimension "d306" = 55
  constraint vertical L0
  constraint horizontal L1
  constraint vertical L2
  constraint horizontal L3
  constraint vertical L4
  constraint horizontal L5
  constraint vertical L6
  constraint horizontal L7
  constraint vertical L10
  constraint horizontal L8
  constraint vertical L9
  constraint horizontal L11
  constraint coincident L2 L11.start
  constraint perpendicular L0 L12
  constraint horizontal L13
  constraint vertical L14
  constraint horizontal L15
  constraint vertical L16
  measures "d284" distance of L2.end L0.start
  measures "d285" distance of L2.end L1.end
  measures "d286" distance of L3.start L3.end
  measures "d287" distance of L3.start L5.end
  measures "d289" distance of L7.start L7.end
  measures "d290" distance of L7.start L8.end
  measures "d294" diameter of A0
  measures "d296" diameter of A1
  measures "d306" distance of L13.start L15.end
extrude "Extrude2" add sketch "Sketch2" along normal blind 5 contours L203 L204 L211 L217 L218 L219 L220 L221 L222 L223 L224 L230 L241 L242 L248 L249 L250 L257 L260 L266 L270 makes body 1
extrude "Extrude3" add sketch "Sketch2" along normal blind 160 separate body contours L5 L6 L7 L8 L11 L12 L13 L14 L16 L17 L18 L19 | L20 L24 L25 L26 L27 L48 L50 L51 | L65 L77 L78 L82 L85 L87 L88 L89 | L166 L167 L168 L171 L172 L173 L175 L183 L184 L185 L190 L195 makes body 2 at (130, 53.3333, -21.6667) makes body 3 at (190, 106.6667, -19) makes body 4 at (100, 53.3333, -21.6667) makes body 5 at (230, 106.6667, -19)
extrude "Extrude4" add sketch "Sketch2" along normal blind 10 separate body contours L0 L1 L2 L3 L4 L28 L29 L30 L33 L34 L37 L38 L39 L40 L41 L42 L43 L44 L45 L46 L47 makes body 6
extrude "Extrude6" add sketch "Sketch6" along normal blind 10 separate body contours L0 L1 L2 L12 makes body 7
move_body "Move1" bodies 1 to x (1, 0, 0) y (0, 1, 0) z (0, 0, 1) at (0, 0, -110)
move_body "Move2" bodies 5 4 3 2 to x (0, -1, 0) y (1, 0, 0) z (0, 0, 1) at (230, 230, 30)
move_body "Move3" bodies 2 3 4 to x (1, 0, 0) y (0, 1, 0) z (0, 0, 1) at (10, 0, 0)
move_body "Move4" bodies 4 to x (1, 0, 0) y (0, 1, 0) z (0, 0, 1) at (-10, -130, 140)
move_body "Move5" bodies 2 to x (1, 0, 0) y (0, 1, 0) z (0, 0, 1) at (-180, -100, 0)
move_body "Move6" bodies 3 to x (1, 0, 0) y (0, 1, 0) z (0, 0, 1) at (-170, -40, 140)
move_body "Move7" bodies 1 6 to x (1, 0, 0) y (0, 1, 0) z (0, 0, 1) at (-10, 0, 30)
extrude "Extrude7" add sketch "Sketch6" along normal blind 80 separate body contours L3 L4 L5 L6 | L7 L8 L9 L10 makes body 8 at (-183.3333, 26.6667, 135) makes body 9 at (-183.3333, 26.6667, 160)
move_body "Move8" bodies 9 8 to x (1, 0, 0) y (0, 0, 1) z (0, -1, 0) at (0, 145, 145)
move_body "Move9" bodies 8 to x (1, 0, 0) y (0, 1, 0) z (0, 0, 1) at (0, -20, -90)
move_body "Move10" bodies 9 8 to x (0, 0, 1) y (0, 1, 0) z (-1, 0, 0) at (345, 0, 495)
move_body "Move11" bodies 9 to x (1, 0, 0) y (0, 1, 0) z (0, 0, 1) at (0, 7, 0)
move_body "Move12" bodies 8 to x (1, 0, 0) y (0, 1, 0) z (0, 0, 1) at (0, 2, 0)
move_body "Move13" bodies 1 to x (1, 0, 0) y (0, 1, 0) z (0, 0, 1) at (0, -7.6, 0)
move_body "Move14" bodies 1 to x (1, 0, 0) y (0, 1, 0) z (0, 0, 1) at (0, 8, 0)
move_body "Move15" bodies 2 9 5 8 4 3 to x (1, 0, 0) y (0, 1, 0) z (0, 0, 1) at (0, 8, 0)
move_body "Move16" bodies 3 to x (1, 0, 0) y (0, 1, 0) z (0, 0, 1) at (-5, 0, 0)
move_body "Move17" bodies 8 9 to x (1, 0, 0) y (0, 1, 0) z (0, 0, 1) at (100, 0, -40)
move_body "Move18" bodies 7 to x (0, 0, 1) y (0, 1, 0) z (-1, 0, 0) at (244.8308, 0, 386.0613)
move_body "Move19" bodies 8 7 9 to x (0, 0, 1) y (0, 1, 0) z (-1, 0, 0) at (155, 0, -155)
move_body "Move20" bodies 7 to x (0.707107, 0, 0.707107) y (0, 1, 0) z (-0.707107, 0, 0.707107) at (-76.6011, 0, 114.7111)
